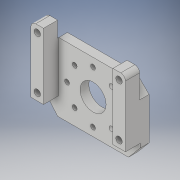
# Autodesk Inventor part: knee_connector_new
Saved by Autodesk Inventor 2018 (Build 220112000, 112)
## iProperties
Created: 2019-04-16
Part Number: knee_connector_new
Material: Generic
Document SubType Name: Modeling
Designer: Jasper
Density: 1 g/cm^3
Appearance: Default
Author: Jasper
Autodesk Inventor part; units mm, degrees
ref_plane "YZ Plane" through (0, 0, 0) normal (1, 0, 0) x (0, 1, 0)
ref_plane "Work Plane1" through (0, 0, -34) normal (0, 0, -1) x (-1, 0, 0)
sketch "Sketch1" plane through (0, 0, -34) normal (0, 0, -1) x (-1, 0, 0)
  line L0 (-15, 14.5) -> (-11.5, 14.5) projected
  line L1 (-15, 14.5) -> (-20.1, 8.5) projected
  line L2 (-20.1, 8.5) -> (-20.1, -44.6) projected
  line L3 (-20.1, -44.6) -> (-15, -50.6) projected
  line L4 (-15, -50.6) -> (15, -50.6) projected
  line L5 (15, -50.6) -> (20.1, -44.6) projected
  line L6 (20.1, -44.6) -> (20.1, 8.5) projected
  line L7 (20.1, 8.5) -> (15, 14.5) projected
  line L8 (11.5, 14.5) -> (15, 14.5) projected
  arc A0 (14.5, 11.5) -> (11.5, 14.5) centre (11.5, 11.5) ccw projected
  line L9 (14.5, -42) -> (14.5, 11.5) projected
  arc A1 (11.5, -45) -> (14.5, -42) centre (11.5, -42) ccw projected
  line L10 (-11.5, -45) -> (11.5, -45) projected
  arc A2 (-14.5, -42) -> (-11.5, -45) centre (-11.5, -42) ccw projected
  line L11 (-14.5, 11.5) -> (-14.5, -42) projected
  arc A3 (-11.5, 14.5) -> (-14.5, 11.5) centre (-11.5, 11.5) ccw projected
  circle A4 centre (17.3, 4) radius 1.35 projected
  circle A5 centre (17.3, -18) radius 1.35 projected
  circle A6 centre (17.3, -40) radius 1.35 projected
  circle A7 centre (11, -47.8) radius 1.35 projected
  circle A8 centre (-17.3, 4) radius 1.35 projected
  circle A9 centre (-17.3, -18) radius 1.35 projected
  circle A10 centre (-17.3, -40) radius 1.35 projected
  circle A11 centre (-11, -47.8) radius 1.35 projected
  line L12 (-20.1, -18.05) -> (-20.1, -15.05)
  line L13 (-20.1, -18.05) -> (-17.1, -18.05) construction
  line L14 (-20.1, -18.05) -> (-20.1, -44.6)
  line L15 (-20.1, -44.6) -> (-15, -50.6)
  line L16 (-15, -50.6) -> (15, -50.6)
  line L17 (15, -50.6) -> (20.1, -44.6)
  line L18 (20.1, -44.6) -> (20.1, -18.05)
  line L19 (20.1, -18.05) -> (20.1, -15.05)
  line L20 (20.1, -18.05) -> (23.1, -18.05) construction
  line L21 (20.1, -15.05) -> (-20.1, -15.05)
  point P0 (0, 0)
  dimension "d0" = 3
  dimension "d1" = 90
  dimension "d2" = 3
  dimension "d3" = 90
  constraints: 20 end point, 5 collinear, 3 perpendicular, 2 horizontal, 2 midpoint
  measures "d0" distance of L12.start L12.end
  measures "d1" angle of L13 L12
  measures "d2" distance of L18.end L19.end
  measures "d3" angle of L20 L19
ref_plane "Work Plane2" through (-19.4786, -19.4786, -43.1) normal (0, 0, -1) x (-0.6619, 0.7496, 0)
extrude "Extrusion1" add sketch "Sketch1" along normal blind 10 contours L21 L11 A2 L10 A1 L9 L6 L5 L4 L3 L2 | L21 L9 A1 L10 A2 L11 | A7 | A11
sketch "Sketch2" plane through (0, 0, -34) normal (0, 0, 1) x (1, 0, 0)
  line L0 (15, 14.5) -> (11.5, 14.5) projected
  line L1 (15, 14.5) -> (20.1, 8.5) projected
  line L2 (20.1, 8.5) -> (20.1, -44.6) projected
  line L3 (20.1, -44.6) -> (15, -50.6) projected
  line L4 (15, -50.6) -> (-15, -50.6) projected
  line L5 (-15, -50.6) -> (-20.1, -44.6) projected
  line L6 (-20.1, -44.6) -> (-20.1, 8.5) projected
  line L7 (-20.1, 8.5) -> (-15, 14.5) projected
  line L8 (-11.5, 14.5) -> (-15, 14.5) projected
  arc A0 (-11.5, 14.5) -> (-14.5, 11.5) centre (-11.5, 11.5) ccw projected
  line L9 (-14.5, -42) -> (-14.5, 11.5) projected
  arc A1 (-14.5, -42) -> (-11.5, -45) centre (-11.5, -42) ccw projected
  line L10 (11.5, -45) -> (-11.5, -45) projected
  arc A2 (11.5, -45) -> (14.5, -42) centre (11.5, -42) ccw projected
  line L11 (14.5, 11.5) -> (14.5, -42) projected
  arc A3 (14.5, 11.5) -> (11.5, 14.5) centre (11.5, 11.5) ccw projected
  circle A4 centre (-17.3, 4) radius 1.35 projected
  circle A5 centre (-17.3, -18) radius 1.35 projected
  circle A6 centre (-17.3, -40) radius 1.35 projected
  circle A7 centre (-11, -47.8) radius 1.35 projected
  circle A8 centre (17.3, 4) radius 1.35 projected
  circle A9 centre (17.3, -18) radius 1.35 projected
  circle A10 centre (17.3, -40) radius 1.35 projected
  circle A11 centre (11, -47.8) radius 1.35 projected
  line L12 (-20.1, -15.05) -> (20.1, -15.05) projected
  line L13 (14.5, -15.05) -> (14.7, -15.05)
  line L14 (14.7, -15.05) -> (14.7, -40)
  line L15 (14.7, -15.05) -> (39.65, -15.05) construction
  line L16 (14.7, -40) -> (14.7, -43)
  line L17 (14.7, -43) -> (-14.7, -43)
  line L18 (-14.7, -43) -> (-14.7, -15.05)
  line L19 (-14.7, -15.05) -> (14.7, -15.05)
  line L20 (14.7, -15.05) -> (14.7, -43)
  point P0 (0, 0)
  dimension "d6" = 0.2
  dimension "d8" = 90
  dimension "d9" = 3
  dimension "d10" = 29.4
  dimension "d11" = 27.95
  constraints: 16 end point, 5 point on line, 2 horizontal, 2 parallel, 2 perpendicular
  measures "d6" distance of L13.start L13.end
  measures "d8" angle of L14 L15
  measures "d9" distance of L14.end L16.end
  measures "d10" distance of L18.end L19.end
  measures "d11" distance between parallel lines of L17 L12
extrude "Extrusion2" cut sketch "Sketch2" against normal blind 6.3 contours L12 L14 L16 L17 A2 L11 | L11 A2 L17 A1 L9 L12 | L9 A1 L17 L18 L12
sketch "Sketch4" plane through (0, 0, -34) normal (0, 0, 1) x (1, 0, 0)
  line L0 (-14.7, -43) -> (-14.7, -15.05) projected
  line L1 (-14.7, -43) -> (-20.1, -43)
  line L2 (-20.1, -44.6) -> (-20.1, -15.05) projected
  line L3 (-20.1, -43) -> (20.1, -43)
  line L4 (20.1, -43) -> (20.1, -50.6)
  line L5 (20.1, -50.6) -> (-20.1, -50.6)
  line L6 (-20.1, -50.6) -> (-20.1, -43)
  point P0 (0, 0)
  dimension "d14" = 7.6
  dimension "d15" = 40.2
  constraints: 10 end point, 2 horizontal, 2 parallel, 1 perpendicular, 1 point on line
  measures "d14" distance between parallel lines of L5 L3
  measures "d15" distance of L4.end L5.end
extrude "Extrusion3" cut sketch "Sketch4" against normal blind 6.3
sketch "Sketch5" plane through (0, 0, -44) normal (0, 0, -1) x (-1, 0, 0)
  line L0 (-20.1, -15.05) -> (-20.1, -44.6) projected
  line L1 (-20.1, -15.05) -> (-20.1, -36.05)
  line L2 (-20.1, -15.05) -> (0.9, -15.05) construction
  line L3 (-20.1, -36.05) -> (0, -36.05)
  line L4 (-20.1, -36.05) -> (0, -36.05) construction
  circle A0 centre (0, -36.05) radius 5.5
  line L5 (0, -36.05) -> (0, -47.05)
  line L6 (0, -36.05) -> (11, -36.05) construction
  circle A1 centre (0, -47.05) radius 1.025
  circle A2 centre (7.7782, -43.8282) radius 1.025
  circle A3 centre (11, -36.05) radius 1.025
  circle A4 centre (7.7782, -28.2718) radius 1.025
  circle A5 centre (0, -25.05) radius 1.025
  circle A6 centre (-7.7782, -28.2718) radius 1.025
  circle A7 centre (-11, -36.05) radius 1.025
  circle A8 centre (-7.7782, -43.8282) radius 1.025
  point P0 (0, 0)
  dimension "d18" = 21
  dimension "d19" = 90
  dimension "d23" = 20.1
  dimension "d24" = 0
  dimension "d25" = 11
  dimension "d26" = 11
  dimension "d27" = 90
  dimension "d28" = 2.05
  dimension "d31" = 360
  constraints: 12 end point, 9 centre point, 4 horizontal, 3 equal length, 2 coincident, 1 collinear, 1 perpendicular, 17 other
  measures "d18" distance of L0.start L1.end
  measures "d19" angle of L1 L2
  measures "d23" distance of L1.end L3.end
  measures "d24" distance between parallel lines of L3 L4
  measures "d25" diameter of A0
  measures "d26" distance of L5.start L5.end
  measures "d27" angle of L5 L6
  measures "d28" diameter of A1
extrude "Extrusion4" cut sketch "Sketch5" against normal up to surface (3.7 mm away)
sketch "Sketch7" plane through (0, 0, -44) normal (0, 0, -1) x (-1, 0, 0)
  circle A0 centre (-7.7782, -43.8282) radius 1.025 construction
  circle A1 centre (0, -36.05) radius 5.5 construction
  circle A2 centre (-11, -36.05) radius 1.025 construction
  circle A3 centre (0, -25.05) radius 1.025 construction
  circle A4 centre (11, -36.05) radius 1.025 construction
  circle A5 centre (0, -47.05) radius 1.025 construction
  circle A6 centre (7.7782, -43.8282) radius 1.025 construction
  circle A7 centre (7.7782, -28.2718) radius 1.025 construction
  circle A8 centre (-7.7782, -28.2718) radius 1.025 construction
  circle A9 centre (-17.3, -40) radius 1.35 construction
  circle A10 centre (-17.3, -18) radius 1.35 construction
  circle A11 centre (17.3, -40) radius 1.35 construction
  circle A12 centre (17.3, -18) radius 1.35 construction
  line L0 (-20.1, -44.6) -> (-15, -50.6) construction
  line L1 (-15, -50.6) -> (15, -50.6) construction
  line L2 (15, -50.6) -> (20.1, -44.6) construction
  line L3 (20.1, -44.6) -> (20.1, -15.05) construction
  line L4 (20.1, -15.05) -> (-20.1, -15.05) construction
  line L5 (-20.1, -15.05) -> (-20.1, -44.6) construction
  line L6 (-20.1, -15.05) -> (-20.1, -27.05)
  line L7 (-20.1, -15.05) -> (-20.1, -44.6) construction
  line L8 (-20.1, -15.05) -> (-8.1, -15.05)
  line L9 (0, -15.05) -> (0, -21.5) construction
  line L10 (0, -21.5) -> (20.1, -21.5) construction
  line L11 (0, -21.5) -> (20.1, -21.5) construction
  line L12 (0, -21.5) -> (-20.1, -21.5) construction
  line L13 (0, -21.5) -> (20.1, -21.5) construction
  line L14 (-20.1, -27.05) -> (-14.55, -21.5)
  line L15 (-20.1, -27.05) -> (-12.2511, -27.05) construction
  line L16 (0, -15.05) -> (20.1, -15.05)
  line L17 (20.1, -15.05) -> (20.1, -27.05)
  line L18 (20.1, -27.05) -> (14.55, -21.5)
  line L19 (14.55, -21.5) -> (-14.55, -21.5)
  line L20 (-14.7, -15.05) -> (-20.1, -15.05) projected
  line L21 (-20.1, -15.05) -> (20.1, -15.05)
  point P0 (0, 0)
  dimension "d40" = 12
  dimension "d41" = 90
  dimension "d42" = 6.45
  dimension "d43" = 20.1
  dimension "d44" = 0
  dimension "d45" = 20.1
  dimension "d46" = 180
  dimension "d47" = 45
  dimension "d48" = 12
  dimension "d49" = 90
  dimension "d50" = 45
  constraints: 28 end point, 7 horizontal, 4 collinear, 4 equal length, 2 point on line, 1 midpoint, 1 vertical
  measures "d40" distance of L4.end L6.end
  measures "d41" angle of L6 L8
  measures "d42" distance of L9.start L9.end
  measures "d43" distance of L9.end L10.end
  measures "d44" distance between parallel lines of L10 L11
  measures "d45" distance of L9.end L12.end
  measures "d46" angle of L12 L13
  measures "d47" angle of L15 L14
  measures "d48" distance of L3.end L17.end
  measures "d49" angle of L16 L17
  measures "d50" angle of L17 L18
extrude "Extrusion5" cut sketch "Sketch7" against normal blind 4
sketch "Sketch10" plane through (20.1, -44.6, -40.3) normal (1, 0, 0) x (0, 0, -1)
  line L0 (3.7, 17.55) -> (-0.3, 17.55) construction
  line L1 (-0.3, 17.55) -> (-0.3, 29.55) construction
  line L2 (-6.3, 29.55) -> (-0.3, 29.55) construction
  line L3 (-6.3, 29.55) -> (-6.3, 1.6) construction
  line L4 (-6.3, 1.6) -> (0, 1.6) construction
  line L5 (0, 1.6) -> (0, 0) construction
  line L6 (0, 0) -> (3.7, 0) construction
  line L7 (3.7, 17.55) -> (3.7, 0) construction
  line L8 (0, 0) -> (0, -6) construction
  line L9 (0, -6) -> (3.7, -6) construction
  line L10 (3.7, 0) -> (3.7, -6) construction
  line L11 (0, 0) -> (3.7, 0) construction
  line L12 (-6.3, 29.55) -> (-0.3, 29.55) projected
  line L13 (-6.3, 29.55) -> (3.7, 29.55)
  line L14 (3.7, 29.55) -> (3.7, -6)
  line L15 (3.7, -6) -> (-6.3, -6)
  line L16 (-6.3, -6) -> (-6.3, 29.55)
  point P0 (-40.3, 44.6)
  constraints: 8 end point, 2 parallel, 1 horizontal, 1 perpendicular
sketch "Sketch12" plane through (-20.1, -44.6, -44) normal (-1, 0, 0) x (0, 0, 1)
  line L0 (4, 17.55) -> (0, 17.55) construction
  line L1 (0, 0) -> (0, 17.55) construction
  line L2 (3.7, 0) -> (0, 0) construction
  line L3 (3.7, 0) -> (3.7, 1.6) construction
  line L4 (3.7, 1.6) -> (10, 1.6) construction
  line L5 (10, 1.6) -> (10, 29.55) construction
  line L6 (10, 29.55) -> (4, 29.55) construction
  line L7 (4, 29.55) -> (4, 17.55) construction
  line L8 (3.7, -6) -> (3.7, 0) construction
  line L9 (3.7, 0) -> (0, 0) construction
  line L10 (0, -6) -> (0, 0) construction
  line L11 (3.7, -6) -> (0, -6) construction
  line L12 (10, 29.55) -> (4, 29.55) projected
  line L13 (3.7, -6) -> (0, -6) projected
  line L14 (10, 29.55) -> (0, 29.55)
  line L15 (0, 29.55) -> (0, -6)
  line L16 (0, -6) -> (10, -6)
  line L17 (10, -6) -> (10, 29.55)
  point P0 (44, 44.6)
  constraints: 8 end point, 2 parallel, 1 horizontal, 1 perpendicular
extrude "Extrusion8" cut sketch "Sketch10" against normal blind 0.1
extrude "Extrusion9" cut sketch "Sketch12" against normal blind 0.1
fillet "Fillet2" radius 2 2 edges at (-20, -15.05, -37) (20, -15.05, -37)
body "Solid1"
